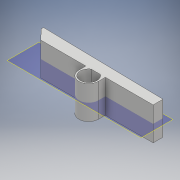
# Autodesk Inventor part: dropper
Saved by Autodesk Inventor 2018 (Build 220112000, 112)
## iProperties
Created: 2017-12-25
Part Number: dropper
Material: Generic
Document SubType Name: Modeling
Designer: mzhang
Density: 1 g/cm^3
Appearance: Default
Author: mzhang
Autodesk Inventor part; units mm, degrees
ref_plane "YZ Plane" through (0, 0, 0) normal (1, 0, 0) x (0, 1, 0)
ref_plane "XZ Plane" through (0, 0, 0) normal (0, 1, 0) x (-1, 0, 0)
ref_plane "XY Plane" through (0, 0, 0) normal (0, 0, 1) x (1, 0, 0)
sketch "Sketch1" plane through (0, 0, 0) normal (0, 0, 1) x (1, 0, 0)
  arc A0 (-1.6733, 2.55) -> (1.6733, 2.55) centre (0, 0) ccw
  line L0 (1.6733, 2.55) -> (-1.6733, 2.55)
  line L1 (0, 2.55) -> (-20, 2.55)
  line L2 (-20, 2.55) -> (-20, 3.55)
  line L3 (-20, 3.55) -> (0, 3.55)
  line L4 (0, 3.55) -> (0, 2.55)
  line L5 (0, 2.55) -> (20, 2.55)
  line L6 (20, 2.55) -> (20, 3.55)
  line L7 (20, 3.55) -> (0, 3.55)
  line L8 (0, 3.55) -> (0, 2.55)
  arc A1 (-3.55, 0) -> (3.55, 0) centre (0, 0) ccw
  line L9 (-3.55, 0) -> (-3.55, 2.55)
  line L10 (3.55, 0) -> (3.55, 2.55)
  dimension "d1" = 6.1
  dimension "d3" = 20
  dimension "d4" = 1
  dimension "d5" = 20
  constraints: 22 end point, 5 parallel, 4 point on circle, 4 point on line, 3 perpendicular, 2 centre point, 2 coincident, 2 horizontal, 2 tangent, 1 midpoint
  measures "d1" diameter of A0
  measures "d3" distance of L3.end L2.end
  measures "d4" distance of L1.end L2.end
  measures "d5" distance of L3.end L6.end
extrude "Extrusion1" add sketch "Sketch1" along normal blind 10
extrude "Extrusion2" cut sketch "Sketch1" along normal blind 10 contours L0 A0
sketch "Sketch3" plane through (0, 0, 10) normal (0, 0, 1) x (1, 0, 0)
  line L0 (20, 3.55) -> (-20, 3.55) projected
  line L1 (-20, 3.55) -> (-23.4721, 7.0221)
  line L2 (-20, 3.55) -> (-15.0898, 3.55) construction
  line L3 (-20, 2.55) -> (-3.55, 2.55) projected
  line L4 (-20, 2.55) -> (-23.4721, 6.1479)
  line L5 (-23.4721, 6.1479) -> (-23.4721, 7.0221)
  line L6 (3.55, 2.55) -> (20, 2.55) projected
  line L7 (20, 2.55) -> (21, 2.55)
  line L8 (21, 2.55) -> (21, 6.1479)
  line L9 (21, 6.1479) -> (20, 6.1479)
  line L10 (20, 6.1479) -> (20, 2.55)
  line L11 (-20, 3.55) -> (-20, 2.55) projected
  line L12 (-20, 3.55) -> (-20, 2.55)
  point P0 (0, 0)
  dimension "d10" = 135
  dimension "d11" = 5
  dimension "d12" = 1
  constraints: 18 end point, 4 equal length, 2 horizontal, 2 perpendicular
  measures "d10" angle of L2 L1
  measures "d11" distance of L3.start L4.end
  measures "d12" distance of L9.end L8.end
extrude "Extrusion3" add sketch "Sketch3" against normal up to surface (10 mm away)
sketch "Sketch4" plane through (0, 0, 10) normal (0, 0, 1) x (1, 0, 0)
  line L0 (-23.4721, 7.0221) -> (-20, 3.55) projected
  line L1 (21, 2.55) -> (21, 6.1479) projected
  line L2 (-23.4721, 7.0221) -> (21, 6.1479)
  line L3 (21, 6.1479) -> (21, 2.55)
  line L4 (-20, 2.55) -> (-3.55, 2.55) projected
  line L5 (21, 2.55) -> (-20, 2.55)
  line L6 (-23.4721, 6.1479) -> (-20, 2.55) projected
  line L7 (-20, 2.55) -> (-23.4721, 6.1479)
  line L8 (-20, 3.55) -> (-23.4721, 7.0221) projected
  line L9 (-23.4721, 6.1479) -> (-23.4721, 7.0221)
  point P0 (0, 0)
  constraints: 10 end point, 2 collinear, 2 perpendicular
extrude "Extrusion4" add sketch "Sketch4" along normal blind 1
ref_plane "Work Plane1" through (0, 0, 5) normal (0, 0, -1) x (-1, 0, 0)
mirror "Mirror1" about plane through (0, 0, 5) normal (0, 0, -1) of "Extrusion4"
sketch "Sketch5" plane through (0, 0, 0) normal (0, 0, -1) x (-1, 0, 0)
  line L0 (3.55, 2.55) -> (1.6733, 2.55) projected
  arc A0 (-1.6733, 2.55) -> (1.6733, 2.55) centre (0, 0) ccw projected
  line L1 (-1.6733, 2.55) -> (-3.55, 2.55) projected
  line L2 (-3.55, 0) -> (-3.55, 2.55) projected
  arc A1 (-3.55, 0) -> (3.55, 0) centre (0, 0) ccw projected
  line L3 (3.55, 2.55) -> (3.55, 0) projected
extrude "Extrusion5" add sketch "Sketch5" along normal up to surface (1 mm away)
sketch "Sketch6" plane through (0, 0, 10) normal (0, 0, 1) x (1, 0, 0)
  line L0 (-1.6733, 2.55) -> (-3.55, 2.55) projected
  line L1 (-3.55, 2.55) -> (-3.55, 0) projected
  arc A0 (-3.55, 0) -> (3.55, 0) centre (0, 0) ccw projected
  line L2 (3.55, 0) -> (3.55, 2.55) projected
  line L3 (3.55, 2.55) -> (1.6733, 2.55) projected
  arc A1 (-1.6733, 2.55) -> (1.6733, 2.55) centre (0, 0) ccw projected
extrude "Extrusion6" add sketch "Sketch6" along normal up to surface (1 mm away)
body "Solid1"
